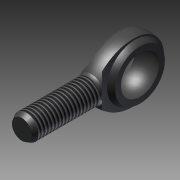
# Autodesk Inventor part: POS 14ECBody
Saved by Autodesk Inventor 2011 SP1 (Build 150282100, 282)
## iProperties
Created: 2017-09-07
Part Number: POS 14ECBody
Catalog Web Link: www.cadenas.de
Description: re_with_m_thread_BO-
Vendor: IKO
Document SubType Name: Modeling
Designer: psAdmin
Manufacturer: IKO
Mass: 11.7681 g
Surface Area: 53.3275 cm^2
Volume: 11.7681 cm^3
Density: 1 g/cm^3
Category: PARTsolutions
Company: IKO
Title: POS 14ECBody
Author: Cadenas PARTsolutions
PSOL_IDENT_0: {$CADENAS_DATA\23d-libs\iko\iko_bearings\pillobals\maintenance_free_type\re_with_m_thread_bo.prj},17
PSOL_IDENT_1: 9 {VTYP=3D},{NB=POS 14ECBody},{LINA=POS 14ECBody},{NN=re_with_m_thread_BO},{DATE=13.10.2016 10:02:14
PSOL_IDENT_2: },{GEOMDATE=04.12.2007 14:31:00},{VERSION=},{LINEID=80},{LINESUBID=-1},{WBVAR=}  {NB=POS 14ECBody},{
PSOL_IDENT_3: LINA=POS 14ECBody},{KT=DUMMY},{IDNR=},{STDRT=14},{ORDER=POS 14EC},{MASS=126.0},{SD=14},{G=M14x2},{ND
PSOL_IDENT_4: M=14},{P1=2.00},{SD2=34},{C1=13.50},{B=19},{SD1=16.9},{SL2=77},{SH=60},{SL1=36},{SR1=0.2},{SDK=25.40
PSOL_IDENT_5: 0},{D4=28.1059},{C2=7.5001},{C3=7.5},{AA=0.0000},{BB=0},{R2=4.0},{R3=26.0},{R4=16.7669},{C=60},{LL6=
PSOL_IDENT_6: 38.25},{LL7=41.5},{LL8=2.4249},{LL9=0.0000},{LL10=0.0000},{LL11=75.6000},{CD=33600},{CS=17200},{SL10=
PSOL_IDENT_7: 0.0000},{G1=14},{GG1=11.835},{PP=2.00},{BL=2},{SC=1},{DBL=25.40}
NN: re_with_m_thread_BO
NB: POS 14ECBody
NBSYN: $ORDER.Body
LINA: POS 14ECBody
STDRT: 14
ORDER: POS 14EC
MASS: 126.0
SD: 14
G: M14x2
NDM: 14
P1: 2.00
SD2: 34
C1: 13.50
B: 19
SD1: 16.9
SL2: 77
SH: 60
SL1: 36
SR1: 0.2
SDK: 25.400
D4: 28.1059
C2: 7.5001
C3: 7.5
AA: 0.0000
BB: 0
R2: 4.0
R3: 26.0
R4: 16.7669
C: 60
LL6: 38.25
LL7: 41.5
LL8: 2.4249
LL9: 0.0000
LL10: 0.0000
LL11: 75.6000
CD: 33600
CS: 17200
SL10: 0.0000
G1: 14
GG1: 11.835
PP: 2.00
BL: 2
SC: 1
DBL: 25.40
SUPPLIER: IKO
ARTICLENO: POS 14ECBody
BOMINFO: POS 14ECBody
CREATOR: CADENAS GmbH
Autodesk Inventor part; units mm, degrees
ref_plane "YZ Plane" through (0, 0, 0) normal (1, 0, 0) x (0, 1, 0)
ref_plane "XZ Plane" through (0, 0, 0) normal (0, 1, 0) x (-1, 0, 0)
ref_plane "XY Plane" through (0, 0, 0) normal (0, 0, 1) x (1, 0, 0)
sketch "Sketch_4" plane through (0, 0, 0) normal (0, 0, 1) x (1, 0, 0)
  line L0 (0, -36) -> (0, 41)
  arc A0 (17, 24) -> (0, 41) centre (0, 24) ccw
  arc A1 (7.5441, 3.1836) -> (17, 24) centre (-8.9892, 23.2497) ccw
  arc A2 (7.5441, 3.1836) -> (7, 1.1694) centre (11, 1.1694) ccw
  line L1 (7, 1.1694) -> (7, -33.5751)
  line L2 (7, -33.5751) -> (5.6, -36)
  line L3 (5.6, -36) -> (0, -36)
  line L4 (0, -36) -> (0, 41)
  constraints: 10 end point, 6 point on circle, 3 centre point
revolve "Revolution1" add sketch "Sketch_4" angle 360 about axis through (0, -36, 0) along (0, -1, 0)
thread "Thread1" size "M14x2" class "6g" standard "ISO Metric profile" full length
sketch "Sketch_5" plane through (0, 0, 0) normal (0, 0, 1) x (1, 0, 0)
  line L0 (-25.5, 42.8) -> (-25.5, -39.6)
  line L1 (-25.5, -39.6) -> (25.5, -39.6)
  line L2 (25.5, -39.6) -> (25.5, 42.8)
  line L3 (25.5, 42.8) -> (-25.5, 42.8)
  line L4 (-7, 2.25) -> (-7, -36)
  line L5 (-7, -36) -> (7, -36)
  line L6 (7, -36) -> (7, 2.25)
  line L7 (7, 2.25) -> (3.7501, 5.5)
  line L8 (3.7501, 5.5) -> (3.7501, 41)
  line L9 (3.7501, 41) -> (-3.7501, 41)
  line L10 (-3.7501, 41) -> (-3.7501, 5.5)
  line L11 (-3.7501, 5.5) -> (-7, 2.25)
  constraints: 24 end point
extrude "Extrusion1" cut sketch "Sketch_5" along normal mid plane 34
sketch "Sketch_6" plane through (0, 0, 0) normal (0, 0, 1) x (1, 0, 0)
  line L0 (6.75, 24) -> (-6.75, 24)
  line L1 (-6.75, 24) -> (-6.75, 38.053)
  arc A0 (-3.7501, 39.6) -> (-6.75, 38.053) centre (2.3958, 24.0001) ccw
  line L2 (-3.7501, 39.6) -> (3.7501, 39.6)
  arc A1 (6.75, 38.053) -> (3.7501, 39.6) centre (-2.3958, 24.0001) ccw
  line L3 (6.75, 38.053) -> (6.75, 24)
  line L4 (6.75, 24) -> (-6.75, 24)
  constraints: 10 end point, 4 point on circle, 2 centre point
revolve "Revolution2" add sketch "Sketch_6" angle 360 about axis through (6.75, 24, 0) along (1, 0, 0)
sketch "Sketch_7" plane through (0, 0, 0) normal (0, 0, 1) x (1, 0, 0)
  line L0 (12.7, 24) -> (-12.7, 24)
  arc A0 (12.7, 24) -> (-12.7, 24) centre (0, 24) ccw
  line L1 (12.7, 24) -> (-12.7, 24)
  constraints: 4 end point, 2 point on circle, 1 centre point
revolve "Revolution3" cut sketch "Sketch_7" angle 360 about axis through (12.7, 24, 0) along (1, 0, 0)
ref_plane "IP_1_BO_XY" through (0, 24, 0) normal (1, 0, 0) x (0, 0, -1)
ref_plane "IP_1_BO_YZ" through (0, 24, 0) normal (0, 0, -1) x (0, 1, 0)
ref_plane "IP_1_BO_ZX" through (0, 24, 0) normal (0, 1, 0) x (1, 0, 0)
body "Solid1"
